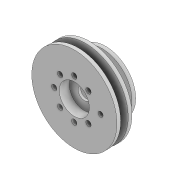
# Autodesk Inventor part: Motor_pulley
Saved by Autodesk Inventor 2022 (Build 260153000, 153)
## iProperties
Created: 2022-07-09
Part Number: Motor_pulley
Material: Generic
Document SubType Name: Modeling
Designer: dell
Density: 1 g/cm^3
Appearance: Default
Author: dell
Autodesk Inventor part; units mm, degrees
ref_plane "YZ Plane" through (0, 0, 0) normal (1, 0, 0) x (0, 1, 0)
ref_plane "XZ Plane" through (0, 0, 0) normal (0, 1, 0) x (-1, 0, 0)
ref_plane "XY Plane" through (0, 0, 0) normal (0, 0, 1) x (1, 0, 0)
sketch "Sketch1" plane through (0, 0, 0) normal (1, 0, 0) x (0, 1, 0)
  line L0 (0, 3) -> (14, 3)
  line L1 (14, 3) -> (14, -3)
  line L2 (14, -3) -> (0, -3)
  line L3 (0, -3) -> (0, 3)
  line L4 (0, -4.2) -> (0, 4.2) projected
  line L5 (14, 1.5) -> (14, -1.5)
  line L6 (14, -1.5) -> (10, -1.5)
  line L7 (10, -1.5) -> (10, 1.5)
  line L8 (10, 1.5) -> (14, 1.5)
  point P0 (0, 0)
  dimension "d0" = 6
  dimension "d1" = 3
  dimension "d2" = 14
  dimension "d4" = 1.5
  dimension "d5" = 1.5
  dimension "d19" = 4
  constraints: 16 end point, 4 parallel, 2 perpendicular, 2 point on line, 1 horizontal, 1 midpoint, 1 vertical
  measures "d0" distance of L2.end L0.start
  measures "d1" distance from line of point (0, 0) L0
  measures "d2" distance between parallel lines of L1 L3
  measures "d4" distance from line of L0 L5.start
  measures "d5" distance of L1.end L5.end
  measures "d19" distance of L5.end L6.end
revolve "Revolution1" add sketch "Sketch1" angle 360 about axis through (0, 0, -10) along (0, 0, 1) contours L0 L1 L8 L7 L6 L2 L3
sketch "Sketch2" plane through (0, 0, -3) normal (0, 0, -1) x (-1, 0, 0)
  circle A0 centre (0, 8) radius 1.05
  circle A1 centre (0, 0) radius 4.5
  dimension "d7" = 2.1
  dimension "d8" = 8
  dimension "d9" = 9
  constraints: 2 centre point, 1 coincident
  measures "d7" diameter of A0
  measures "d8" distance of point (0, 0) A0.centre
  measures "d9" diameter of A1
extrude "Extrusion1" cut sketch "Sketch2" against normal blind 100
pattern_circular "Circular Pattern1" count 8 over 360 about axis through (0, 0, -10) along (0, 0, 1) of "Extrusion1"
sketch "Sketch3" plane through (0, 0, -3) normal (0, 0, -1) x (-1, 0, 0)
  circle A0 centre (-10.5, 0) radius 1
  point P0 (0, 0)
  dimension "d15" = 2
  dimension "d16" = 10.5
  constraints: 1 centre point
  measures "d15" diameter of A0
  measures "d16" distance of point (0, 0) A0.centre
extrude "Extrusion2" cut sketch "Sketch3" against normal blind 100
sketch "Sketch4" plane through (0, 0, -3) normal (0, 0, -1) x (-1, 0, 0)
  circle A0 centre (-10.5, 0) radius 1 projected
  circle A1 centre (-8, 0) radius 1.05 projected
  circle A2 centre (0, -8) radius 1.05 projected
  circle A3 centre (8, 0) radius 1.05 projected
  circle A4 centre (5.6569, 5.6569) radius 1.05 projected
  circle A5 centre (5.6569, -5.6569) radius 1.05 projected
  circle A6 centre (-5.6569, -5.6569) radius 1.05 projected
  circle A7 centre (-5.6569, 5.6569) radius 1.05 projected
  circle A8 centre (0, 0) radius 4.5 projected
  circle A9 centre (0, 8) radius 1.05 projected
  circle A10 centre (0, 0) radius 14 projected
  arc A11 (-9.9643, -0.8444) -> (-9.9643, 0.8444) centre (0, 0) ccw projected
  arc A12 (-9.9643, -0.8444) -> (-9.9643, 0.8444) centre (0, 0) ccw projected
  circle A13 centre (0, 0) radius 5
  point P0 (-9.9643, -0.8444)
  point P1 (-9.9643, 0.8444)
  dimension "d24" = 10
  constraints: 1 centre point, 1 coincident
  measures "d24" diameter of A13
extrude "Extrusion3" add sketch "Sketch4" along normal blind 5 and the other way blind 2 contours A8 | A13
sketch "Sketch9" plane through (0, 0, -1) normal (0, 0, 1) x (1, 0, 0)
  circle A0 centre (0, 0) radius 2.5
  dimension "d37" = 5
  constraints: 1 centre point, 1 coincident
  measures "d37" diameter of A0
extrude "Extrusion8" cut sketch "Sketch9" against normal blind 1
sketch "Sketch7" plane through (0, 0, -8) normal (0, 0, -1) x (-1, 0, 0)
  circle A0 centre (-5, 0) radius 1
  circle A1 centre (0, 0) radius 5 projected
  dimension "d31" = 2
  constraints: 1 centre point, 1 horizontal alignment, 1 other
  measures "d31" diameter of A0
extrude "Extrusion6" cut sketch "Sketch7" against normal blind 4 contours A0 A1 | A1 A0 picked at (-4.6592, 0) picked at (-5.3259, 0)
sketch "Sketch8" plane through (0, 0, -8) normal (0, 0, -1) x (-1, 0, 0)
  circle A0 centre (0, 0) radius 9
  arc A1 (-4.9, -0.995) -> (-4.9, 0.995) centre (-5, 0) ccw projected
  arc A2 (-4.9, -0.995) -> (-4.9, 0.995) centre (-5, 0) ccw projected
  circle A3 centre (-5, 0) radius 1
  arc A4 (-4.9, -0.995) -> (-4.9, 0.995) centre (0, 0) ccw projected
  point P0 (-4.3889, 0.9938)
  point P1 (-4.3889, -0.9938)
  dimension "d34" = 18
  constraints: 2 centre point, 2 coincident
  measures "d34" diameter of A0
extrude "Extrusion7" add sketch "Sketch8" along normal blind 1.5 contours A0 | A1 A4
sketch "Sketch11" plane through (0, 0, -3) normal (0, 0, -1) x (-1, 0, 0)
  circle A0 centre (-10.5, 0) radius 1 projected
  circle A1 centre (-8, 0) radius 1.05 projected
  circle A2 centre (0, -8) radius 1.05 projected
  circle A3 centre (8, 0) radius 1.05 projected
  circle A4 centre (5.6569, 5.6569) radius 1.05 projected
  circle A5 centre (5.6569, -5.6569) radius 1.05 projected
  circle A6 centre (-5.6569, -5.6569) radius 1.05 projected
  circle A7 centre (-5.6569, 5.6569) radius 1.05 projected
  circle A8 centre (0, 8) radius 1.05 projected
  circle A9 centre (0, 0) radius 14 projected
  circle A10 centre (-5.6569, 5.6569) radius 2
  circle A11 centre (0, 8) radius 2
  circle A12 centre (5.6569, 5.6569) radius 2
  circle A13 centre (8, 0) radius 2
  circle A14 centre (5.6569, -5.6569) radius 2
  circle A15 centre (0, -8) radius 2
  circle A16 centre (-5.6569, -5.6569) radius 2
  line L0 (-7.5, 3) -> (-18.9706, 3)
  line L1 (-18.9706, 3) -> (-18.9706, -3)
  line L2 (-18.9706, -3) -> (-7.5, -3)
  line L3 (-7.5, -3) -> (-7.5, 3)
  circle A17 centre (0, 0) radius 5 projected
  circle A18 centre (0, 0) radius 11.5
  point P0 (-4.3889, -0.9938)
  point P1 (-4.3889, 0.9938)
  point P2 (-7.5, -0.9233)
  point P3 (-13.6748, -3)
  point P4 (-13.6748, 3)
  point P5 (-7.5, 0.9233)
  point P6 (-11.1018, 3)
  point P7 (-11.1018, -3)
  dimension "d44" = 4
  dimension "d45" = 4
  dimension "d46" = 4
  dimension "d47" = 4
  dimension "d48" = 4
  dimension "d49" = 4
  dimension "d50" = 4
  dimension "d51" = 3
  dimension "d52" = 3
  dimension "d53" = 3
  dimension "d58" = 23
  constraints: 8 centre point, 8 coincident, 8 end point, 2 parallel, 1 horizontal, 1 perpendicular
  measures "d44" diameter of A10
  measures "d45" diameter of A11
  measures "d46" diameter of A12
  measures "d47" diameter of A13
  measures "d48" diameter of A14
  measures "d49" diameter of A15
  measures "d50" diameter of A16
  measures "d51" distance from line of point (0, 0) L0
  measures "d52" distance from line of point (0, 0) L2
  measures "d53" distance from line of A0.centre L3
  measures "d58" diameter of A18
extrude "Extrusion10" add sketch "Sketch11" along normal blind 1.6 contours A18 L2 L3 A1 L0 | A17 picked at (-9.5578, -3.8503)
extrude "Extrusion11" add sketch "Sketch11" against normal blind 6 contours L3 A1 | A1 L3
thicken "Thicken1" operation add thickness 3 both sides no extend neighbours yes toward (0.0804666, 0.9967573, 0) faces at (1.1265, 13.9546, 2)
thicken "Thicken2" operation add thickness 3 both sides no extend neighbours yes toward (0.0804666, 0.9967573, 0) faces at (1.1265, 13.9546, -2.5)
thicken "Thicken3" operation add thickness 3 both sides no extend neighbours yes toward (-0.9967573, -0.0804666, 0) faces at (-8.9708, -0.7242, -9)
fillet "Fillet1" radius 1 2 edges at (-11.5, 0, -4.6) (-11.5, 0, -3)
thicken "Thicken4" operation add thickness 1.5 both sides no extend neighbours yes toward (-0.9870503, -0.1604113, 0) faces at (-4.4417, -0.7219, 1.6667)
sketch "Sketch10" plane through (0, 0, -8) normal (0, 0, 1) x (1, 0, 0)
  circle A0 centre (0, 0) radius 24.9442
  constraints: 1 centre point, 1 coincident
body "Solid1"
